ExtraDownPlate v3 (Autodesk Fusion 360 design; units mm, degrees)
Autodesk Fusion 360 part; units mm, degrees
sketch "Sketch1" plane through (0, 0, 0) normal (0, 1, 0) x (1, 0, 0)
  circle A0 centre (0, 0) radius 20.5 construction
  circle A1 centre (0, 0) radius 36.8935
  circle A2 centre (0, 0) radius 23.5
  dimension "d1" = 41
  dimension "d2" = 73.787
  dimension "d3" = 3
  constraint coincident A0.centre A1.centre
  measures "d1" diameter of A0
  measures "d2" diameter of A1
extrude "Extrude1" add sketch "Sketch1" along normal blind 4
